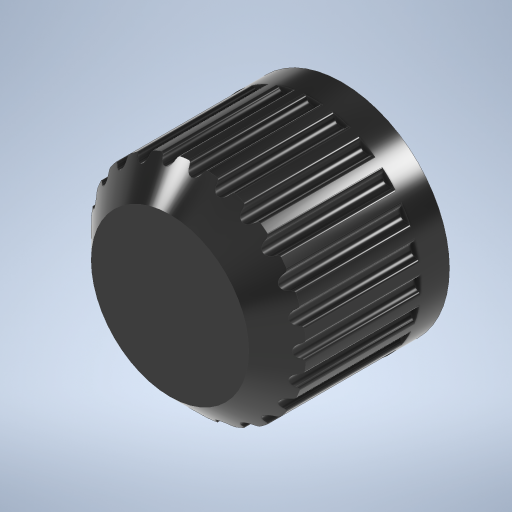
# Autodesk Inventor part: Encder Knob
Saved by Autodesk Inventor 2024 (Build 280153000, 153)
## iProperties
Created: 2025-09-13
Part Number: Encder Knob
Material: Generic
Document SubType Name: Modeling
Designer: Login
Density: 1 g/cm^3
Appearance: Default
Author: Login
Autodesk Inventor part; units mm, degrees
ref_plane "YZ Plane" through (0, 0, 0) normal (1, 0, 0) x (0, 1, 0)
ref_plane "XZ Plane" through (0, 0, 0) normal (0, 1, 0) x (-1, 0, 0)
ref_plane "XY Plane" through (0, 0, 0) normal (0, 0, 1) x (1, 0, 0)
sketch "Sketch1" plane through (0, 0, 0) normal (0, 0, 1) x (1, 0, 0)
  circle A0 centre (0, 0) radius 7.5
  dimension "d0" = 15
  constraints: 1 centre point, 1 coincident
  measures "d0" diameter of A0
extrude "Extrusion1" add sketch "Sketch1" along normal blind 12
chamfer "Chamfer1" distance 2 angle 45 1 edges at (-7.5, 0, 12)
shell "Shell1" thickness 2 removed faces 1 at (-2.141, -0.5635, 0)
sketch "Sketch3" plane through (0, 0, 12) normal (0, 0, 1) x (1, 0, 0)
  circle A0 centre (0, 0) radius 7.5 projected
  circle A1 centre (0, 7.5) radius 0.5
  point P0 (-0.4997, 7.4833)
  point P1 (0.4997, 7.4833)
  dimension "d16" = 1
  dimension "d17" = 0
  constraints: 1 centre point, 2 other
  measures "d16" diameter of A1
  measures "d17" horizontal distance of point (0, 0) A1.centre
extrude "Extrusion3" cut sketch "Sketch3" against normal blind 10 contours A1 A0 picked at (0.0197, 7.3333)
fillet "Fillet2" radius 0.2 2 edges at (-0.4997, 7.4833, 6) (0.4997, 7.4833, 6)
pattern_circular "Circular Pattern2" count 24 over 360 about axis through (0, 0, -10) along (0, 0, 1) of "Extrusion3", "Fillet2"
sketch "Sketch4" plane through (0, 0, 10) normal (0, 0, -1) x (-1, 0, 0)
  circle A0 centre (0, 0) radius 4
  circle A1 centre (0, 0) radius 3
  dimension "d24" = 8
  dimension "d25" = 6
  constraints: 2 centre point, 2 coincident
  measures "d24" diameter of A0
  measures "d25" diameter of A1
extrude "Extrusion4" add sketch "Sketch4" along normal blind 8.5
sketch "Sketch5" plane through (0, 0, 10) normal (0, 0, -1) x (-1, 0, 0)
  circle A0 centre (0, 0) radius 3 projected
  circle A1 centre (0, 0) radius 3
  line L0 (2.5981, 1.5) -> (-2.5981, 1.5)
  dimension "d28" = 4.5
  dimension "d29" = 6
  constraints: 2 end point, 2 point on circle, 1 centre point, 1 coincident, 1 horizontal
  measures "d29" diameter of A1
extrude "Extrusion5" add sketch "Sketch5" along normal blind 6.6 contours L0 A0 picked at (0.7274, 1.6862)
chamfer "Chamfer2" distance 0.5 angle 45 1 edges at (4, 0, 10)
chamfer "Chamfer4" distance 0.5 angle 45 1 edges at (3, 0, 1.5)
chamfer "Chamfer5" distance 1 angle 45 1 edges at (-5.5, 0, 0)
sketch "Sketch6" plane through (0, 0, 0) normal (0, 0, -1) x (-1, 0, 0)
  circle A0 centre (0, 0) radius 3.5 projected
  circle A1 centre (0, 0) radius 6.5 projected
  line L0 (-0.5, 3.5) -> (0.5, 3.5)
  line L1 (0.5, 3.5) -> (0.5, 6.5)
  line L2 (0.5, 6.5) -> (-0.5, 6.5)
  line L3 (-0.5, 6.5) -> (-0.5, 3.5)
  line L4 (-0.5, 3.5) -> (0.5, 6.5) construction
  line L5 (0.5, 3.5) -> (-0.5, 6.5) construction
  point P0 (0, 5)
  point P1 (-0.5, 6.4807)
  point P2 (0.5, 6.4807)
  dimension "d50" = 1
  constraints: 12 end point, 2 midpoint, 2 parallel, 2 tangent, 1 horizontal, 1 perpendicular
  measures "d50" distance of L1.end L2.end
extrude "Extrusion6" add sketch "Sketch6" against normal up to next contours L0 L3 A1 L1 picked at (-0.2778, 4.4971)
pattern_circular "Circular Pattern3" count 5 over 360 about axis through (0, 0, -10) along (0, 0, 1) of "Extrusion6"
sketch "Sketch7" plane through (0, 0, 0) normal (0, 0, -1) x (-1, 0, 0)
  line L0 (0.4, -4) -> (-0.4, -4)
  line L1 (-0.4, -4) -> (-0.4, -2.9732)
  line L2 (-0.4, -2.9732) -> (0.4, -2.9732)
  line L3 (0.4, -2.9732) -> (0.4, -4)
  line L4 (0.4, -4) -> (-0.4, -2.9732) construction
  line L5 (-0.4, -4) -> (0.4, -2.9732) construction
  arc A0 (4.2138, -4.9491) -> (6.3181, 1.5271) centre (0, 0) ccw projected
  line L6 (3.4832, 0.606) -> (6.3181, 1.5271) construction
  line L7 (6.3181, 1.5271) -> (3.9289, 0.7508) construction
  line L8 (4.2138, -4.9491) -> (2.4618, -2.5377) construction
  line L9 (0, 0) -> (6.5959, -2.1431) construction
  line L10 (3.6806, -1.6165) -> (2.7041, -1.2992)
  line L11 (2.7041, -1.2992) -> (2.9513, -0.5384)
  line L12 (2.9513, -0.5384) -> (3.9278, -0.8556)
  line L13 (3.9278, -0.8556) -> (3.6806, -1.6165)
  line L14 (3.6806, -1.6165) -> (2.9513, -0.5384) construction
  line L15 (2.7041, -1.2992) -> (3.9278, -0.8556) construction
  circle A1 centre (0, 0) radius 3 projected
  arc A2 (2.7372, -2.9168) -> (3.9289, 0.7508) centre (0, 0) ccw projected
  arc A3 (-1.9282, -3.5046) -> (1.9282, -3.5046) centre (0, 0) ccw projected
  line L16 (0, 0) -> (0, -3.4866) construction
  line L17 (-3.6806, -1.6165) -> (-2.7041, -1.2992)
  line L18 (-2.7041, -1.2992) -> (-2.9513, -0.5384)
  line L19 (-2.9513, -0.5384) -> (-3.9278, -0.8556)
  line L20 (-3.9278, -0.8556) -> (-3.6806, -1.6165)
  line L21 (-3.6806, -1.6165) -> (-2.9513, -0.5384) construction
  line L22 (-2.7041, -1.2992) -> (-3.9278, -0.8556) construction
  point P0 (3.316, -1.0774)
  point P1 (-3.316, -1.0774)
  point P2 (-2.9513, -0.5384)
  point P3 (0.4, -3.9799)
  point P4 (-0.4, -3.9799)
  point P5 (3.6616, -1.6103)
  point P6 (3.9088, -0.8494)
  dimension "d51" = 0.8
  dimension "d52" = 36
  dimension "d53" = 0.8
  constraints: 42 end point, 6 midpoint, 5 symmetric about line, 4 parallel, 4 point on circle, 2 perpendicular, 2 tangent, 1 collinear, 1 horizontal, 1 point on line
  measures "d51" distance of L1.end L2.end
  measures "d52" angle of L6 L9
  measures "d53" distance of L10.end L11.end
extrude "Extrusion7" cut sketch "Sketch7" against normal blind 4 contours A3 L1 A1 L3 | A1 L12 A2 L10 | L17 L20 L19 A1
fillet "Fillet3" radius 0.4 6 edges at (-3.43, -0.6939, 4) (-3.1828, -1.4547, 4) (-0.4, -3.4766, 4) (0.4, -3.4766, 4) (3.1828, -1.4547, 4) (3.43, -0.6939, 4)
chamfer "Chamfer6" distance 2.95 distance2 1.5 1 edges at (2.0572, -2.8316, 0) measured on face at (-4.3252, 1.2301, 0)
chamfer "Chamfer7" distance 2.95 distance2 1.5 1 edges at (3.3287, 1.0816, 0) measured on face at (-4.3252, 1.2301, 0)
chamfer "Chamfer8" distance 2.95 distance2 1.5 1 edges at (0, 3.5, 0) measured on face at (-4.3252, 1.2301, 0)
chamfer "Chamfer9" distance 2.95 distance2 1.5 1 edges at (-3.3287, 1.0816, 0) measured on face at (-4.3252, 1.2301, 0)
chamfer "Chamfer10" distance 2.95 distance2 1.5 1 edges at (-2.0572, -2.8316, 0) measured on face at (-2.7761, -3.5374, 0)
body "Solid1"
